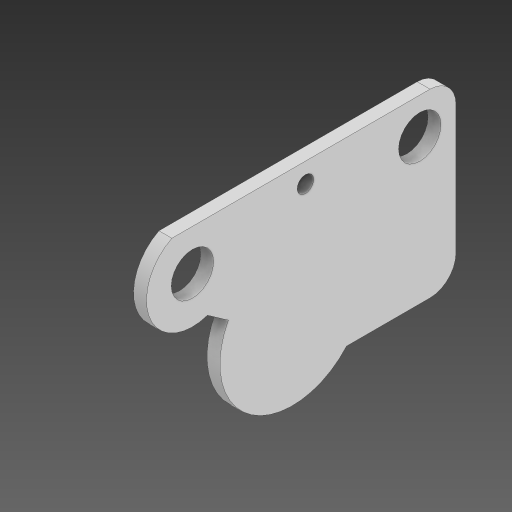
# Autodesk Inventor part: koleso_rig
Saved by Autodesk Inventor 2023 (Build 270158000, 158)
## iProperties
Created: 2025-05-23
Part Number: koleso_rig
Material: Типовые
Document SubType Name: Sheet Metal
Designer: daa
Density: 1 g/cm^3
Appearance: По умолчанию
Sheet Metal Rule: По умолчанию
Author: daa
Autodesk Inventor part; units mm, degrees
ref_plane "YZ Plane" through (0, 0, 0) normal (1, 0, 0) x (0, 1, 0)
ref_plane "XZ Plane" through (0, 0, 0) normal (0, 1, 0) x (-1, 0, 0)
ref_plane "XY Plane" through (0, 0, 0) normal (0, 0, 1) x (1, 0, 0)
sketch "Эскиз1" plane through (0, 0, 0) normal (1, 0, 0) x (0, 1, 0)
  circle A0 centre (24.7003, 51.0226) radius 4.1
  arc A1 (32.6573, 54.9999) -> (16.2986, 48.0999) centre (24.7003, 51.0226) ccw
  line L0 (32.6573, 54.9999) -> (32.6573, 4.9999)
  circle A2 centre (25.6573, 7) radius 4.1
  circle A3 centre (2.6573, 5) radius 1.6
  arc A4 (27.6247, 0) -> (32.6573, 4.9999) centre (27.6573, 4.9999) ccw
  circle A5 centre (6.9066, 31.6862) radius 14
  line L1 (16.2986, 48.0999) -> (13.4489, 44.0635)
  arc A6 (13.4489, 44.0635) -> (-2.2631, 21.1071) centre (6.9066, 31.6862) ccw
  circle A7 centre (28.8003, 29.1433) radius 1.6
  line L2 (27.6247, 0) -> (2.6573, 0)
  line L3 (-2.3427, 5) -> (-2.3427, 21.1767)
  arc A8 (-2.3427, 5) -> (2.6573, 0) centre (2.6573, 5) ccw
  line L4 (6.9066, 31.6862) -> (25.6573, 7)
  point P0 (0, 0)
  point P1 (9.1696, 29.0795)
  point P2 (-2.3427, 0)
  dimension "d9" = 8.2
  dimension "d86" = 8.2
  dimension "d87" = 3.2
  dimension "d92" = 5
  dimension "d111" = 50
  dimension "d132" = 28
  dimension "d145" = 3.2
  dimension "d159" = 35
  dimension "d160" = 5
  dimension "d161" = 5
  dimension "d167" = 8.8956
  dimension "d171" = 4.0364
  dimension "d173" = 21.1767
  dimension "d191" = 31
  dimension "d192" = 7
  dimension "d193" = 7
  constraints: 11 point on circle, 10 end point, 9 centre point, 3 concentric, 3 tangent, 2 coincident, 2 point on line, 2 vertical, 1 horizontal
  measures "d9" diameter of A0
  measures "d86" diameter of A2
  measures "d87" diameter of A3
  measures "d92" radius of A4
  measures "d111" distance of L0.start L0.end
  measures "d132" diameter of A5
  measures "d145" diameter of A7
  measures "d159" distance from line of L0 point (-2.343, 0)
  measures "d160" radius of A8
  measures "d161" distance from line of L3 A3.centre
  measures "d167" radius of A1
  measures "d171" vertical distance of L1.start L1.end
  measures "d173" vertical distance of L3.end L2.end
  measures "d191" distance of L4.start L4.end
  measures "d192" distance from line of L0 L4.end
  measures "d193" distance from line of L2 A2.centre
extrude "Выдавливание1" add sketch "Эскиз1" along normal blind 2.5
sketch "Эскиз6" plane through (2.5, 0, 0) normal (1, 0, 0) x (0, 0, -1)
  circle A0 centre (-4.9913, 2.6582) radius 1.6
  circle A1 centre (-4.9913, 2.6582) radius 3.1
  circle A2 centre (-29.0488, 28.7734) radius 1.6
  circle A3 centre (-29.0488, 28.7734) radius 2.6
  point P0 (0, 0)
  dimension "d180" = 3.2
  dimension "d181" = 6.2
  dimension "d182" = 3.2
  dimension "d183" = 5.2
  constraints: 4 centre point, 2 coincident
  measures "d180" diameter of A0
  measures "d181" diameter of A1
  measures "d182" diameter of A2
  measures "d183" diameter of A3
extrude "Выдавливание6" add sketch "Эскиз6" against normal blind 17.5 contours A0 | A1
sketch "Эскиз7" plane through (-15, 2.6582, 4.9913) normal (-1, 0, 0) x (0, 0, 1)
  circle A0 centre (0, 0) radius 1.95
  point P0 (-4.9913, -2.6582)
  dimension "d188" = 3.9
  constraints: 1 centre point
  measures "d188" diameter of A0
extrude "Выдавливание7" cut sketch "Эскиз7" against normal blind 4.5
equation "\"Радиус_гибки\" = Толщина"
equation "\"Ширина_просечки\" = Толщина"
equation "\"Глубина_просечки\" = 0.5 * Толщина"
equation "\"Размер_просечки\" = 4 * Толщина"
equation "\"Мин_остаток\" = 2 * Толщина"
equation "\"Радиус_перехода\" = Радиус_гибки"
equation "\"Радиус_Якоби\" = Радиус_гибки"
equation "\"Размер_зазора\" = Толщина"
equation "\"Толщина\" = 3.048"
